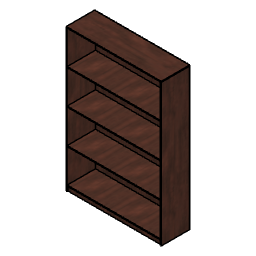
Bookshelf v2 (Autodesk Fusion 360 design; units mm, degrees)
Autodesk Fusion 360 part; units mm, degrees
sketch "Sketch1" plane through (0, 0, 0) normal (0, 0, 1) x (1, 0, 0) in component "Backboard"
  line L0 (500, 750) -> (-500, 750)
  line L1 (-500, 750) -> (-500, -750)
  line L2 (-500, -750) -> (500, -750)
  line L3 (500, -750) -> (500, 750)
  line L4 (500, 750) -> (-500, -750) construction
  line L5 (-500, 750) -> (500, -750) construction
  dimension "d1" = 1000
  dimension "d2" = 1500
  constraint horizontal L0
  constraint perpendicular L0 L1
  constraint parallel L0 L2
  constraint parallel L1 L3
  constraint coincident L4 origin
  constraint coincident L5 origin
  measures "d1" distance of L1.end L2.end
  measures "d2" distance of L0.end L1.end
extrude "Extrude1" add sketch "Sketch1" along normal blind 2.5 makes body 1 in component "Backboard"
sketch "Sketch1 (2)" plane through (0, 0, 0) normal (0, 1, 0) x (1, 0, 0) in component "TopPlank"
  line L0 (0, 0) -> (1000, 0)
  line L1 (1000, 0) -> (1000, 297.5)
  line L2 (1000, 297.5) -> (0, 297.5)
  line L3 (0, 297.5) -> (0, 0)
  dimension "d5" = 1000
  dimension "d6" = 297.5
  constraint horizontal L0
  constraint vertical L1
  constraint horizontal L2
  constraint vertical L3
  constraint coincident L0.start L3.end
  measures "d5" distance of L0.start L0.end
  measures "d6" distance of L0.start L2.end
extrude "Extrude1'" add sketch "Sketch1 (2)" along normal blind 10 separate body makes body 2 in component "TopPlank"
sketch "Sketch1 (3)" plane through (0, 0, 0) normal (1, 0, 0) x (0, 0, -1) in component "SidePanel"
  line L0 (0, 0) -> (297.5, 0)
  line L1 (297.5, 0) -> (297.5, 1490)
  line L2 (297.5, 1490) -> (0, 1490)
  line L3 (0, 1490) -> (0, 0)
  dimension "d13" = 297.5
  dimension "d14" = 1490
  constraint horizontal L0
  constraint vertical L1
  constraint horizontal L2
  constraint vertical L3
  constraint coincident L0.start L3.end
  measures "d13" distance of L0.start L0.end
  measures "d14" distance of L0.start L2.end
extrude "Extrude1''" add sketch "Sketch1 (3)" along normal blind 10 separate body makes body 3 in component "SidePanel"
sketch "Sketch1 (4)" plane through (0, 0, 0) normal (0, 1, 0) x (1, 0, 0) in component "Shelf"
  line L0 (490, 148.75) -> (-490, 148.75)
  line L1 (-490, 148.75) -> (-490, -148.75)
  line L2 (-490, -148.75) -> (490, -148.75)
  line L3 (490, -148.75) -> (490, 148.75)
  line L4 (490, 148.75) -> (-490, -148.75) construction
  line L5 (-490, 148.75) -> (490, -148.75) construction
  dimension "d29" = 980
  dimension "d30" = 297.5
  constraint horizontal L0
  constraint perpendicular L0 L1
  constraint parallel L0 L2
  constraint parallel L1 L3
  constraint coincident L4 origin
  constraint coincident L5 origin
  measures "d29" distance of L1.end L2.end
  measures "d30" distance of L0.end L1.end
extrude "Extrude1'''" add sketch "Sketch1 (4)" along normal blind 10 separate body makes body 4 in component "Shelf"
sketch "Sketch1 (5)" plane through (0, 0, 0) normal (0, 1, 0) x (1, 0, 0) in component "Plinth"
sketch "Sketch2" plane through (0, 0, 0) normal (1, 0, 0) x (0, 0, -1) in component "Plinth"
sketch "Sketch3" plane through (0, 0, 300) normal (0, 0, 1) x (1, 0, 0) in component "Plinth"
  line L0 (490, 740) -> (490, -750)
  line L1 (490, -750) -> (500, -750)
  line L2 (500, -750) -> (500, 740)
  line L3 (500, 740) -> (490, 740)
  line L4 (490, -25) -> (-490, -25)
  line L5 (-490, -25) -> (-490, 25)
  line L6 (-490, 25) -> (490, 25)
  line L7 (490, 25) -> (490, -25)
  line L8 (490, -25) -> (-490, 25) construction
  line L9 (-490, -25) -> (490, 25) construction
  dimension "d39" = 980
  dimension "d40" = 50
  constraint horizontal L4
  constraint perpendicular L4 L5
  constraint parallel L4 L6
  constraint parallel L5 L7
  constraint coincident L8 origin
  constraint coincident L9 origin
  measures "d39" distance of L5.end L6.end
  measures "d40" distance of L4.end L5.end
extrude "Extrude1''''" add sketch "Sketch3" along normal blind 10 separate body contours L0 L4 L5 L6 L7 makes body 5 in component "Plinth"
pattern_linear "00000000-0000-0000-0000-000000000000" [suppressed]
component "Backboard" placed x (1, 0, 0) y (0, 1, 0) z (0, 0, 1) at (0, 0, 0)
component "TopPlank" placed x (1, 0, 0) y (0, 1, 0) z (0, 0, 1) at (-500, 740, 300)
component "SidePanel" placed x (1, 0, 0) y (0, 1, 0) z (0, 0, 1) at (-500, -750, 300)
component "SidePanel" placed x (1, 0, 0) y (0, 1, 0) z (0, 0, 1) at (490, -750, 300)
component "Shelf" placed x (1, 0, 0) y (0, -1, 0) z (0, 0, -1) at (0, -690, 151.25)
component "Plinth" placed x (-1, 0, 0) y (0, 1, 0) z (0, 0, -1) at (0, -725, 590)
component "Shelf" placed x (1, 0, 0) y (0, -1, 0) z (0, 0, -1) at (0, -330, 151.25)
component "Shelf" placed x (1, 0, 0) y (0, -1, 0) z (0, 0, -1) at (0, 30, 151.25)
component "Shelf" placed x (1, 0, 0) y (0, -1, 0) z (0, 0, -1) at (0, 390, 151.25)
equation "d1 = BookcaseWidth"
equation "d2 = BookcaseHeight"
equation "d3 = BackThickness"
equation "d5 = BookcaseWidth"
equation "d6 = BookcaseDepth - BackThickness"
equation "d7 = MainThickness"
equation "d13 = BookcaseDepth - BackThickness"
equation "d14 = BookcaseHeight - MainThickness"
equation "d15 = MainThickness"
equation "MainThickness = 10 mm"
equation "BookcaseWidth = 1000 mm"
equation "BookcaseHeight = 1500 mm"
equation "BookcaseDepth = 300 mm"
equation "d29 = BookcaseWidth - MainThickness * 2"
equation "d30 = BookcaseDepth - BackThickness"
equation "d31 = MainThickness"
equation "BackThickness = 2.5 mm"
equation "d36 = -PlinthHeight"
equation "PlinthHeight = 50 mm"
equation "d39 = BookcaseWidth - MainThickness * 2"
equation "d40 = PlinthHeight"
equation "d41 = MainThickness"
equation "d44 = MainThickness * 2"
equation "VoidHeight = BookcaseHeight - MainThickness - PlinthHeight"
equation "VoidWidth = BookcaseWidth - MainThickness * 2"
equation "d51 = VoidHeight"
